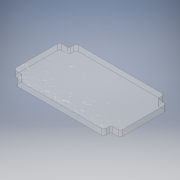
# Autodesk Inventor part: BT702_trajan20_21
Saved by Autodesk Inventor 2022.2 (Build 262287000, 287)
## iProperties
Company: HTBLA Kaindorf
RuleStatus: InUse
Created: 2022-08-21
Part Number: BT702_trajan20_21
Project: Zeichenmaschine_v2
Material: Acryl
Description: Plexi_40x80
Document SubType Name: Modeling
Designer: trajan20
Density: 1.188 g/cm^3
Appearance: Transparent - farblos
Mass: 27.6905 g
Surface Area: 107.282 cm^2
Volume: 23.3085 cm^3
AfterDocNew0: iProperties-Editor_aufrufen
Author: jan
Keywords: 2021
Autodesk Inventor part; units mm, degrees
ref_plane "YZ Plane" through (0, 0, 0) normal (1, 0, 0) x (0, 1, 0)
ref_plane "XZ Plane" through (0, 0, 0) normal (0, 1, 0) x (-1, 0, 0)
ref_plane "XY Plane" through (0, 0, 0) normal (0, 0, 1) x (1, 0, 0)
sketch "Skizze3" plane through (0, 0, 0) normal (0, 0, 1) x (1, 0, 0)
  line L0 (0, 0) -> (-40, 0)
  line L1 (-40, 0) -> (-40, 80)
  line L2 (-40, 80) -> (0, 80)
  line L3 (0, 80) -> (0, 0)
  line L4 (-40, 78.2) -> (-46.3, 78.2)
  line L5 (-46.3, 78.2) -> (-46.3, 40)
  line L6 (-46.3, 40) -> (-40, 40)
  line L7 (-40, 40) -> (-40, 78.2)
  line L8 (-40, 80) -> (-20, 80)
  line L9 (-20, 80) -> (-20, 86.3)
  line L10 (-20, 86.3) -> (-40, 86.3)
  line L11 (-40, 86.3) -> (-40, 80)
  point P0 (-40, 40)
  point P1 (-20, 80)
  dimension "d4" = 80
  dimension "d5" = 40
  dimension "d6" = 6.3
  dimension "d7" = 1.8
  dimension "d8" = 6.3
  constraints: 24 end point, 6 parallel, 3 horizontal, 3 perpendicular, 3 point on line, 2 midpoint
  measures "d4" distance between parallel lines of L2 L0
  measures "d5" distance between parallel lines of L1 L3
  measures "d6" distance between parallel lines of L2 L10
  measures "d7" distance between parallel lines of L2 L4
  measures "d8" distance between parallel lines of L1 L5
extrude "Extrusion3" add sketch "Skizze3" along normal blind 5 contours L0 L1 L2 L3
extrude "Extrusion4" add sketch "Skizze3" along normal blind 5 contours L6 L5 L4 L1 | L2 L11 L10 L9
fillet "Rundung1" radius 2 2 edges at (-46.3, 78.2, 2.5) (-40, 86.3, 2.5)
mirror "Spiegeln1" about plane through (-46.3, 40, 0) normal (0, -1, 0) of "Extrusion4", "Rundung1"
mirror "Spiegeln2" about plane through (-20, 80, 0) normal (1, 0, 0) of "Extrusion4", "Rundung1", "Spiegeln1"
fillet "Rundung2" radius 1.5 4 edges at (0, 78.2, 2.5) (-40, 78.2, 2.5) (-40, 1.8, 2.5) (0, 1.8, 2.5)
equation "\"d8\" = d6"
